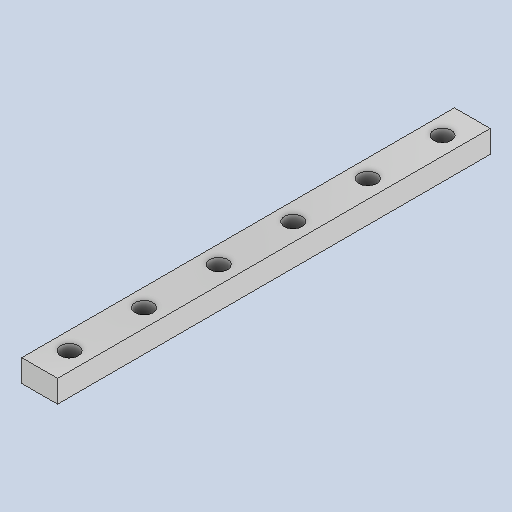
# Autodesk Inventor part: slider
Saved by Autodesk Inventor 2022 (Build 260153070, 153G)
## iProperties
Created: 2022-08-15
Part Number: slider
Material: アルミニウム 6061-AHC
Document SubType Name: Modeling
Designer: zegi
Density: 2.7 g/cm^3
Appearance: アルミニウム - ダーク
Mass: 32.5551 g
Surface Area: 64.4997 cm^2
Volume: 12.0575 cm^3
Author: zegi
Autodesk Inventor part; units mm, degrees
ref_plane "YZ Plane" through (0, 0, 0) normal (1, 0, 0) x (0, 1, 0)
ref_plane "XZ Plane" through (0, 0, 0) normal (0, 1, 0) x (-1, 0, 0)
ref_plane "XY Plane" through (0, 0, 0) normal (0, 0, 1) x (1, 0, 0)
sketch "スケッチ1" plane through (0, 0, 0) normal (0, 0, 1) x (1, 0, 0)
  line L0 (0, 0) -> (12, 0)
  line L1 (12, 0) -> (12, 7.5)
  line L2 (12, 7.5) -> (0, 7.5)
  line L3 (0, 7.5) -> (0, 0)
  dimension "d0" = 12
  dimension "d1" = 7.5
  constraints: 8 end point, 2 parallel, 1 horizontal, 1 perpendicular
  measures "d0" distance of L2.end L1.end
  measures "d1" distance of L1.end L0.end
extrude "押し出し1" add sketch "スケッチ1" along normal blind 145
sketch "スケッチ2" plane through (0, 7.5, 0) normal (0, 1, 0) x (1, 0, 0)
  line L0 (12, -145) -> (0, -145) projected
  line L1 (6, -145) -> (6, 0)
  line L2 (12, 0) -> (0, 0) projected
  point P0 (6, -10)
  point P1 (6, -135)
  point P2 (6, -110)
  point P3 (6, -85)
  point P4 (6, -60)
  point P5 (6, -35)
  dimension "d4" = 10
  dimension "d5" = 10
  dimension "d6" = 25
  dimension "d7" = 25
  dimension "d8" = 25
  dimension "d9" = 25
  dimension "d10" = 25
  constraints: 6 point on line, 2 end point, 2 midpoint
  measures "d4" distance from line of L0 point (6, -135)
  measures "d5" distance from line of L2 point (6, -10)
  measures "d6" distance of point (6, -35) point (6, -10)
  measures "d7" distance of point (6, -60) point (6, -35)
  measures "d8" distance of point (6, -85) point (6, -60)
  measures "d9" distance of point (6, -110) point (6, -85)
  measures "d10" distance of point (6, -135) point (6, -110)
hole "穴1" at (6, 7.5, 10) at (6, 7.5, 135) at (6, 7.5, 110) at (6, 7.5, 85) at (6, 7.5, 60) at (6, 7.5, 35) direction (0, -1, 0) diameter 3.5 end through all
sketch "スケッチ3" plane through (0, 7.5, 0) normal (0, 1, 0) x (1, 0, 0)
  line L0 (12, -145) -> (0, -145)
  line L1 (6, -145) -> (6, 0)
  line L2 (12, 0) -> (0, 0)
  point P0 (6, -10)
  point P1 (6, -135)
  point P2 (6, -110)
  point P3 (6, -85)
  point P4 (6, -60)
  point P5 (6, -35)
  dimension "d18" = 10
  dimension "d19" = 10
  dimension "d20" = 25
  dimension "d21" = 25
  dimension "d22" = 25
  dimension "d23" = 25
  dimension "d24" = 25
  constraints: 6 end point, 6 point on line, 2 midpoint
  measures "d18" distance from line of L0 point (6, -135)
  measures "d19" distance from line of L2 point (6, -10)
  measures "d20" distance of point (6, -35) point (6, -10)
  measures "d21" distance of point (6, -60) point (6, -35)
  measures "d22" distance of point (6, -85) point (6, -60)
  measures "d23" distance of point (6, -110) point (6, -85)
  measures "d24" distance of point (6, -135) point (6, -110)
hole "穴2" at (6, 7.5, 10) at (6, 7.5, 135) at (6, 7.5, 110) at (6, 7.5, 60) at (6, 7.5, 35) at (6, 7.5, 85) direction (0, -1, 0) diameter 6 depth 5
equation "\"d7\" = d6"
equation "\"d8\" = d6"
equation "\"d9\" = d6"
equation "\"d21\" = d20"
equation "\"d22\" = d20"
equation "\"d23\" = d20"
